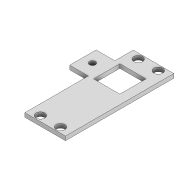
# Autodesk Inventor part: plataforma_nueva
Saved by Autodesk Inventor 2021 (Build 250183000, 183)
## iProperties
Created: 2022-06-07
Part Number: plataforma_nueva
Material: Genérico
Document SubType Name: Modeling
Designer: orgyn
Density: 1 g/cm^3
Appearance: Valor por defecto
Author: orgyn
Autodesk Inventor part; units mm, degrees
ref_plane "YZ Plane" through (0, 0, 0) normal (1, 0, 0) x (0, 1, 0)
ref_plane "XZ Plane" through (0, 0, 0) normal (0, 1, 0) x (-1, 0, 0)
ref_plane "XY Plane" through (0, 0, 0) normal (0, 0, 1) x (1, 0, 0)
sketch "Boceto1" plane through (0, 0, 0) normal (0, 1, 0) x (-1, 0, 0)
  line L0 (0, -30.1) -> (-8.9011, -30.1)
  line L1 (0, -30.1) -> (-10, -30.1)
  line L2 (0, -30.1) -> (10, -30.1)
  line L3 (10, -30.1) -> (10, 23.3)
  line L4 (10, -30.1) -> (63.4, -30.1) construction
  line L5 (10, 23.3) -> (-10, 23.3)
  line L6 (-10, 23.3) -> (-10, -30.1)
  line L7 (-10, 23.3) -> (-10, 20.7)
  line L8 (-10, 20.7) -> (10, 20.7)
  line L9 (0, 20.7) -> (4.95, 20.7)
  line L10 (4.95, 20.7) -> (-4.95, 20.7)
  circle A0 centre (4.95, 20.7) radius 2.2
  circle A1 centre (-4.95, 20.7) radius 2.2
  line L11 (10, 0) -> (5.5615, 0)
  line L12 (-10, -30.1) -> (-10, -27.5)
  circle A2 centre (4.95, -27.5) radius 2.2
  circle A3 centre (-4.95, -27.5) radius 2.2
  circle A4 centre (4.95, 20.7) radius 2.2
  circle A5 centre (-4.95, 20.7) radius 2.2
  line L13 (7.5, -13.5) -> (7.5, -21)
  line L14 (7.5, -21) -> (-5.5, -21)
  line L15 (-5.5, -21) -> (-5.5, -8)
  line L16 (-5.5, -8) -> (7.5, -8)
  line L17 (7.5, -8) -> (7.5, -13.5)
  line L18 (1, -8) -> (1, -21)
  line L19 (-5.5, -14.5) -> (7.5, -14.5)
  line L20 (1, -14.5) -> (14.5, -14.5)
  circle A6 centre (14.5, -14.5) radius 1.5
  line L21 (10, -8) -> (19.2349, -8)
  line L22 (19.2349, -8) -> (19.2349, -21)
  line L23 (19.2349, -21) -> (10, -21)
  point P0 (0, 0)
  dimension "d8" = 53.4
  dimension "d9" = 90
  dimension "d10" = 20
  dimension "d11" = 2.6
  dimension "d12" = 4.95
  dimension "d13" = 9.9
  dimension "d14" = 4.4
  dimension "d15" = 4.4
  dimension "d16" = 2.6
  dimension "d19" = 4.4
  dimension "d20" = 4.4
  dimension "d26" = 13.5
  dimension "d27" = 3
  constraints: 48 end point, 13 point on line, 11 perpendicular, 7 centre point, 5 midpoint, 3 coincident, 3 horizontal
  measures "d8" distance of L2.end L3.end
  measures "d9" angle of L4 L3
  measures "d10" distance of L3.end L5.end
  measures "d11" distance of L5.end L7.end
  measures "d12" distance of L9.start L9.end
  measures "d13" distance of L9.end L10.end
  measures "d14" diameter of A0
  measures "d15" diameter of A1
  measures "d16" distance of L1.end L12.end
  measures "d19" diameter of A4
  measures "d20" diameter of A5
  measures "d26" distance of L20.start L20.end
  measures "d27" diameter of A6
extrude "Extrusión1" add sketch "Boceto1" along normal blind 2 contours L0 L1 L6 L8 A1 A0 L3 L2 | L3 L21 L22 L23 | L6 L5 L3 L8 A0 A1
